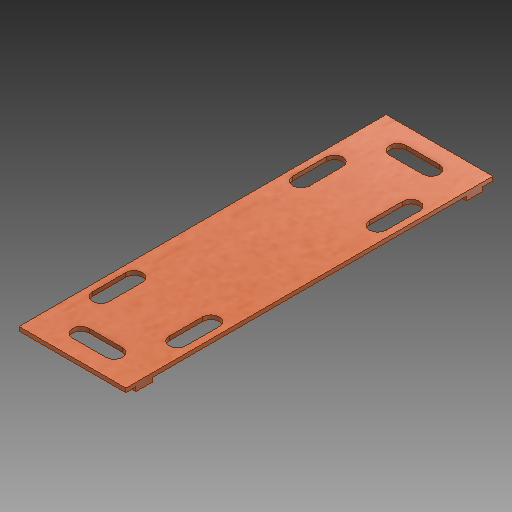
# Autodesk Inventor part: bett_V3_teil2_deckplatte
Saved by Autodesk Inventor 2018 (Build 220112000, 112)
## iProperties
Created: 2020-03-29
Part Number: bett_V3_teil2_deckplatte
Material: Holz (Walnuss)
Document SubType Name: Modeling
Designer: wepet
Density: 0.55 g/cm^3
Appearance: Walnuss - natur - poliert
Description: Sperrholzplatte 12mm - 35x110cm
Mass: 2.11345 g
Surface Area: 68.9828 cm^2
Volume: 3.84263 cm^3
Author: wepet
Autodesk Inventor part; units mm, degrees
ref_plane "YZ Plane" through (0, 0, 0) normal (1, 0, 0) x (0, 1, 0)
ref_plane "XZ Plane" through (0, 0, 0) normal (0, 1, 0) x (-1, 0, 0)
ref_plane "XY Plane" through (0, 0, 0) normal (0, 0, 1) x (1, 0, 0)
sketch "Skizze1" plane through (0, 0, 0) normal (0, 0, 1) x (1, 0, 0)
  line L0 (0, 0) -> (32, 0)
  line L1 (32, 0) -> (32, 110)
  line L2 (32, 110) -> (0, 110)
  line L3 (0, 110) -> (0, 0)
  line L4 (11, 105) -> (21, 105)
  line L5 (21, 105) -> (21, 100) construction
  line L6 (21, 100) -> (11, 100)
  line L7 (11, 100) -> (11, 105) construction
  line L8 (11, 10) -> (21, 10)
  line L9 (21, 10) -> (21, 5) construction
  line L10 (21, 5) -> (11, 5)
  line L11 (11, 5) -> (11, 10) construction
  line L12 (2, 90) -> (7, 90) construction
  line L13 (7, 90) -> (7, 80)
  line L14 (7, 80) -> (2, 80) construction
  line L15 (2, 80) -> (2, 90)
  line L16 (2, 30) -> (7, 30) construction
  line L17 (7, 30) -> (7, 20)
  line L18 (7, 20) -> (2, 20) construction
  line L19 (2, 20) -> (2, 30)
  line L20 (25, 90) -> (30, 90) construction
  line L21 (30, 90) -> (30, 80)
  line L22 (30, 80) -> (25, 80) construction
  line L23 (25, 80) -> (25, 90)
  line L24 (25, 30) -> (30, 30) construction
  line L25 (30, 30) -> (30, 20)
  line L26 (30, 20) -> (25, 20) construction
  line L27 (25, 20) -> (25, 30)
  line L28 (16, 110) -> (16, 0) construction
  line L29 (7, 80) -> (7, 30) construction
  line L30 (0, 55) -> (32, 55) construction
  arc A0 (2, 80) -> (7, 80) centre (4.5, 80) ccw
  arc A1 (7, 90) -> (2, 90) centre (4.5, 90) ccw
  arc A2 (30, 90) -> (25, 90) centre (27.5, 90) ccw
  arc A3 (25, 80) -> (30, 80) centre (27.5, 80) ccw
  arc A4 (21, 5) -> (21, 10) centre (21, 7.5) ccw
  arc A5 (11, 10) -> (11, 5) centre (11, 7.5) ccw
  arc A6 (2, 20) -> (7, 20) centre (4.5, 20) ccw
  arc A7 (25, 20) -> (30, 20) centre (27.5, 20) ccw
  arc A8 (30, 30) -> (25, 30) centre (27.5, 30) ccw
  arc A9 (7, 30) -> (2, 30) centre (4.5, 30) ccw
  arc A10 (21, 100) -> (21, 105) centre (21, 102.5) ccw
  arc A11 (11, 105) -> (11, 100) centre (11, 102.5) ccw
  point P0 (16, 10)
  point P1 (7, 55)
  dimension "d0" = 32
  dimension "d1" = 110
  dimension "d4" = 10
  dimension "d5" = 10
  dimension "d6" = 10
  dimension "d7" = 5
  dimension "d8" = 5
  dimension "d9" = 5
  dimension "d10" = 5
  dimension "d11" = 5
  dimension "d12" = 2
  dimension "d13" = 2
  dimension "d14" = 50
  dimension "d15" = 5
  constraints: 62 end point, 24 point on circle, 18 midpoint, 14 parallel, 12 centre point, 12 point on line, 7 horizontal, 7 perpendicular, 1 collinear, 1 tangent
  measures "d0" distance of L2.end L1.end
  measures "d1" distance of L1.end L0.end
  measures "d4" distance of L9.end L10.end
  measures "d5" distance of L18.end L16.start
  measures "d6" distance of L14.end L12.start
  measures "d7" distance of L17.end L18.end
  measures "d8" distance of L25.end L26.end
  measures "d9" distance of L8.end L9.end
  measures "d10" distance of L4.end L5.end
  measures "d11" distance between parallel lines of L2 L4
  measures "d12" distance between parallel lines of L1 L21
  measures "d13" distance between parallel lines of L3 L15
  measures "d14" distance between parallel lines of L14 L16
  measures "d15" distance between parallel lines of L0 L10
extrude "Extrusion2" add sketch "Skizze1" along normal blind 1.2
sketch "Skizze2" plane through (0, 0, 0) normal (0, 0, -1) x (-1, 0, 0)
  arc A0 (-25, 30) -> (-30, 30) centre (-27.5, 30) ccw construction
  line L0 (-25, 30) -> (-25, 20) construction
  arc A1 (-30, 20) -> (-25, 20) centre (-27.5, 20) ccw construction
  line L1 (-30, 20) -> (-30, 30) construction
  arc A2 (-25, 90) -> (-30, 90) centre (-27.5, 90) ccw construction
  line L2 (-25, 90) -> (-25, 80) construction
  arc A3 (-30, 80) -> (-25, 80) centre (-27.5, 80) ccw construction
  line L3 (-30, 80) -> (-30, 90) construction
  arc A4 (-2, 30) -> (-7, 30) centre (-4.5, 30) ccw construction
  line L4 (-2, 30) -> (-2, 20) construction
  arc A5 (-7, 20) -> (-2, 20) centre (-4.5, 20) ccw construction
  line L5 (-7, 20) -> (-7, 30) construction
  arc A6 (-2, 90) -> (-7, 90) centre (-4.5, 90) ccw construction
  line L6 (-2, 90) -> (-2, 80) construction
  arc A7 (-7, 80) -> (-2, 80) centre (-4.5, 80) ccw construction
  line L7 (-7, 80) -> (-7, 90) construction
  arc A8 (-21, 10) -> (-21, 5) centre (-21, 7.5) ccw construction
  line L8 (-21, 10) -> (-11, 10) construction
  arc A9 (-11, 5) -> (-11, 10) centre (-11, 7.5) ccw construction
  line L9 (-11, 5) -> (-21, 5) construction
  arc A10 (-21, 105) -> (-21, 100) centre (-21, 102.5) ccw construction
  line L10 (-21, 105) -> (-11, 105) construction
  arc A11 (-11, 100) -> (-11, 105) centre (-11, 102.5) ccw construction
  line L11 (-11, 100) -> (-21, 100) construction
  line L12 (0, 0) -> (-32, 0) construction
  line L13 (0, 110) -> (0, 0) construction
  line L14 (-32, 110) -> (0, 110) construction
  line L15 (-32, 0) -> (-32, 110) construction
  line L16 (-32, 3) -> (-27, 3)
  line L17 (-27, 3) -> (-27, 8)
  line L18 (-27, 8) -> (-32, 8)
  line L19 (-32, 8) -> (-32, 3)
  line L20 (0, 3) -> (-5, 3)
  line L21 (-5, 3) -> (-5, 8)
  line L22 (-5, 8) -> (0, 8)
  line L23 (0, 8) -> (0, 3)
  line L24 (0, 102) -> (-5, 102)
  line L25 (-5, 102) -> (-5, 107)
  line L26 (-5, 107) -> (0, 107)
  line L27 (0, 107) -> (0, 102)
  line L28 (-27, 107) -> (-32, 107)
  line L29 (-32, 107) -> (-32, 102)
  line L30 (-32, 102) -> (-27, 102)
  line L31 (-27, 102) -> (-27, 107)
  dimension "d18" = 5
  dimension "d19" = 5
  dimension "d20" = 5
  dimension "d21" = 5
  dimension "d22" = 3
  dimension "d23" = 0
  dimension "d24" = 0
  dimension "d25" = 3
  constraints: 32 end point, 8 parallel, 8 point on line, 4 horizontal, 4 perpendicular
  measures "d18" distance of L18.end L16.start
  measures "d19" distance of L16.start L16.end
  measures "d20" distance of L20.start L20.end
  measures "d21" distance of L28.end L29.end
  measures "d22" distance between parallel lines of L12 L16
  measures "d23" distance between parallel lines of L15 L19
  measures "d24" distance between parallel lines of L13 L23
  measures "d25" distance between parallel lines of L14 L28
extrude "Extrusion3" add sketch "Skizze2" along normal blind 1.2
